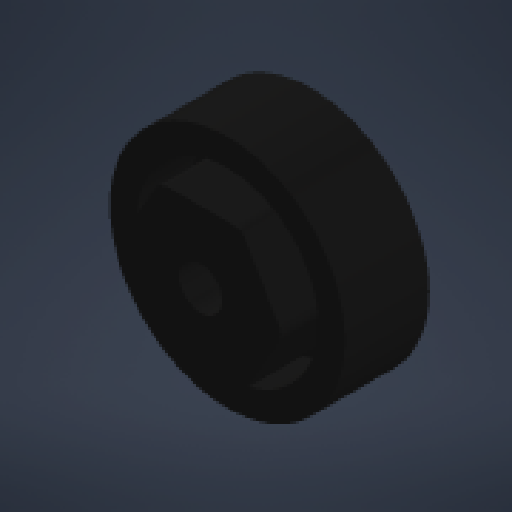
# Autodesk Inventor part: Solenoid Shield
Saved by Autodesk Inventor 2026.1 (Build 301233020, 233B)
## iProperties
Created: 2025-11-08
Part Number: Solenoid Shield
Material: Generic
Document SubType Name: Modeling
Designer: Bahaa
Density: 1 g/cm^3
Appearance: Default
Mass: 1.54071 g
Surface Area: 13.7973 cm^2
Volume: 1.54071 cm^3
Author: Bahaa
Autodesk Inventor part; units mm, degrees
ref_plane "YZ Plane" through (0, 0, 0) normal (1, 0, 0) x (0, 1, 0)
ref_plane "XZ Plane" through (0, 0, 0) normal (0, 1, 0) x (-1, 0, 0)
ref_plane "XY Plane" through (0, 0, 0) normal (0, 0, 1) x (1, 0, 0)
sketch "Sketch1" plane through (0, 0, 0) normal (0, 1, 0) x (-1, 0, 0)
  line L0 (-8.75, 22.75) -> (8.75, 22.75)
  line L1 (8.75, 22.75) -> (8.75, -22.75)
  line L2 (8.75, -22.75) -> (-8.75, -22.75)
  line L3 (-8.75, -22.75) -> (-8.75, 22.75)
  line L4 (-8.75, 22.75) -> (8.75, -22.75) construction
  line L5 (8.75, 22.75) -> (-8.75, -22.75) construction
  line L6 (-1.6021, -2.775) -> (-3.2043, 0)
  line L7 (-3.2043, 0) -> (-1.6021, 2.775)
  line L8 (-1.6021, 2.775) -> (1.6021, 2.775)
  line L9 (1.6021, 2.775) -> (3.2043, 0)
  line L10 (3.2043, 0) -> (1.6021, -2.775)
  line L11 (1.6021, -2.775) -> (-1.6021, -2.775)
  line L12 (6.091, 0) -> (3.0455, 5.275)
  line L13 (3.0455, 5.275) -> (-3.0455, 5.275)
  line L14 (-3.0455, 5.275) -> (-6.091, 0)
  line L15 (-6.091, 0) -> (-3.0455, -5.275)
  line L16 (-3.0455, -5.275) -> (3.0455, -5.275)
  line L17 (3.0455, -5.275) -> (6.091, 0)
  line L18 (6.75, -20.75) -> (6.75, 20.75)
  line L19 (6.75, 20.75) -> (-6.75, 20.75)
  line L20 (-6.75, 20.75) -> (-6.75, -20.75)
  line L21 (-6.75, -20.75) -> (6.75, -20.75)
  circle A0 centre (0, 0) radius 1.6
  circle A1 centre (0, 0) radius 8.75
  circle A2 centre (0, 0) radius 6.75
  dimension "d0" = 17.5
  dimension "d1" = 45.5
  dimension "d2" = 5.55
  dimension "d8" = 2.5
  dimension "d9" = 2
  dimension "d11" = 3.2
  dimension "d14" = 17.5
  dimension "d15" = 2
  constraints: 44 end point, 5 parallel, 3 centre point, 3 coincident, 2 midpoint, 2 perpendicular, 1 horizontal, 21 other
  measures "d0" distance of L1.end L2.end
  measures "d1" distance of L0.end L1.end
  measures "d2" distance between parallel lines of L11 L8
  measures "d8" distance between parallel lines of L9 L12
  measures "d9" distance between parallel lines of L1 L18
  measures "d11" diameter of A0
  measures "d14" diameter of A1
  measures "d15" radial gap between concentric circles of A1 A2
extrude "Extrusion1" add sketch "Sketch1" along normal blind 6.9 contours A1 L20 | A1 L18 | A1 L18 A2 L20 | L20 A2 L18 A1 | A2 | L6 L7 L8 L9 L10 L11 | L17 L16 L15 L14 L13 L12 | A0
extrude "Extrusion5" add sketch "Sketch1" against normal blind 2 contours L6 L7 L8 L9 L10 L11 | L17 L16 L15 L14 L13 L12
extrude "Extrusion2" cut sketch "Sketch1" along normal blind 4 contours A2 | L6 L7 L8 L9 L10 L11 | A0
fillet "Fillet1" radius 1 6 edges at (6.091, 1, 0) (-3.0455, 1, 5.275) (3.0455, 1, -5.275) (-3.0455, 1, -5.275) (-6.091, 1, 0) (3.0455, 1, 5.275)
fillet "Fillet2" [suppressed]
equation "\"d14\" = d0"
body "Solid1"
